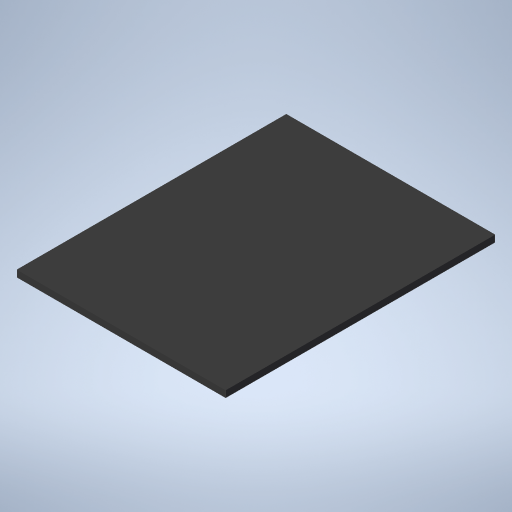
# Autodesk Inventor part: CapRS3
Saved by Autodesk Inventor 2024.3 (Build 283343000, 343)
## iProperties
Created: 2025-06-19
Part Number: CapRS3
Material: Generic
Document SubType Name: Modeling
Designer: ajclo
Density: 1 g/cm^3
Appearance: Default
Author: ajclo
Autodesk Inventor part; units mm, degrees
ref_plane "YZ Plane" through (0, 0, 0) normal (1, 0, 0) x (0, 1, 0)
ref_plane "XZ Plane" through (0, 0, 0) normal (0, 1, 0) x (-1, 0, 0)
ref_plane "XY Plane" through (0, 0, 0) normal (0, 0, 1) x (1, 0, 0)
sketch "Sketch1" plane through (0, 0, 0) normal (0, 1, 0) x (-1, 0, 0)
  line L0 (0, 0) -> (93, 0)
  line L1 (93, 0) -> (93, -120)
  line L2 (93, -120) -> (0, -120)
  line L3 (0, -120) -> (0, 0)
  line L4 (93, -120) -> (55, -120)
  line L5 (93, -116.5) -> (93, -120)
  line L6 (93, 0) -> (55, 0)
  line L7 (93, -3.5) -> (93, 0)
  line L8 (93, -42) -> (93, -112)
  point P0 (46.5, 0)
  dimension "d0" = 120
  dimension "d1" = 93
  constraints: 18 end point, 3 horizontal, 2 parallel, 1 midpoint, 1 perpendicular, 1 point on line
  measures "d0" distance of L0.end L1.end
  measures "d1" distance of L1.end L2.end
extrude "Extrusion1" add sketch "Sketch1" along normal blind 3
body "Solid1"
